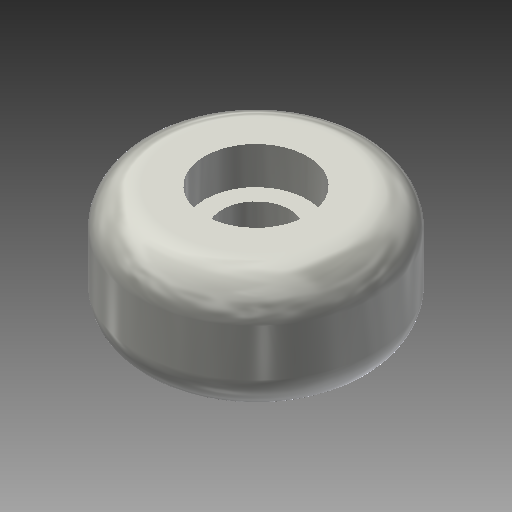
# Autodesk Inventor part: Ruota
Saved by Autodesk Inventor 2019 (Build 230136000, 136)
## iProperties
Created: 2011-10-08
Part Number: Ruota
Document SubType Name: Modeling
Designer: Stefano
Density: 1 g/cm^3
Material: 一般
Appearance: 滑らか - 象牙色
Mass: 41.2872 g
Surface Area: 83.2529 cm^2
Volume: 41.2872 cm^3
Author: Stefano
Autodesk Inventor part; units mm, degrees
ref_plane "YZ Plane" through (0, 0, 0) normal (1, 0, 0) x (0, 1, 0)
ref_plane "XZ Plane" through (0, 0, 0) normal (0, 1, 0) x (-1, 0, 0)
ref_plane "XY Plane" through (0, 0, 0) normal (0, 0, 1) x (1, 0, 0)
sketch "Schizzo1" plane through (0, 0, 0) normal (0, 0, 1) x (1, 0, 0)
  line L0 (0, 0) -> (0, 14.5631) construction
  line L1 (0, 0) -> (7.25, 0) construction
  line L2 (7.25, 10) -> (11, 10)
  line L3 (11, 10) -> (11, 18)
  line L4 (11, 18) -> (25.5, 18)
  line L5 (7.25, 10) -> (7.25, 5)
  line L6 (0, 10) -> (7.25, 10) construction
  line L7 (7.25, 0) -> (11, 0)
  line L8 (11, 0) -> (11, -8)
  line L9 (11, -8) -> (25.5, -8)
  line L10 (7.25, 0) -> (7.25, 5)
  line L11 (7.25, 10) -> (7.25, 5)
  line L12 (25.5, -8) -> (25.5, 18)
  dimension "d0" = 7.25
  dimension "d1" = 10
  dimension "d2" = 11
  dimension "d3" = 8
  dimension "d4" = 25.5
  constraints: 26 end point, 2 perpendicular, 1 parallel, 1 vertical
  measures "d0" distance of L0.start L1.end
  measures "d1" distance of L1.end L2.start
  measures "d2" distance from line of L0 L2.end
  measures "d3" distance of L2.end L3.end
  measures "d4" distance from line of L0 L4.end
revolve "Rivoluzione2" add sketch "Schizzo1" angle 360 about axis through (0, 0, 0) along (0, 1, 0)
fillet "Raccordo2" radius 8 2 edges at (-25.5, 18, 0) (-25.5, -8, 0)
